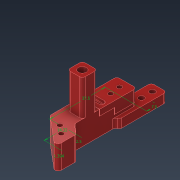
# Autodesk Inventor part: CH_01_0025_end_switch_mount
Saved by Autodesk Inventor 2022.3 (Build 263350030, 350C)
## iProperties
Created: 2022-03-07
Part Number: CH_01_0025_end_switch_mount
Material: Generic
Document SubType Name: Modeling
Designer: Tomasz Krakowski
Density: 1 g/cm^3
Appearance: Czerwona
Mass: 3.3096 g
Surface Area: 18.0709 cm^2
Volume: 3.3096 cm^3
Author: Tomasz Krakowski
Autodesk Inventor part; units mm, degrees
ref_plane "YZ Plane" through (0, 0, 0) normal (1, 0, 0) x (0, 1, 0)
ref_plane "XZ Plane" through (0, 0, 0) normal (0, 1, 0) x (-1, 0, 0)
ref_plane "XY Plane" through (0, 0, 0) normal (0, 0, 1) x (1, 0, 0)
sketch "Sketch2" plane through (0, 0, 0) normal (0, 1, 0) x (-1, 0, 0)
  line L0 (-10, 10) -> (-10, -10)
  line L1 (-10, -10) -> (10, -10)
  line L2 (10, -10) -> (10, -6.782)
  line L3 (10, -6.782) -> (-10, 10)
  line L4 (0, 0) -> (0, -10) construction
  line L5 (0, 0) -> (-10, 0) construction
  dimension "d7" = 20
  dimension "d8" = 20
  dimension "d15" = 50
  constraints: 12 end point, 4 perpendicular, 2 midpoint, 1 vertical
  measures "d7" distance of L0.end L1.end
  measures "d8" distance from line of L1 L0.start
  measures "d15" angle of L0 L3
extrude "Extrusion2" add sketch "Sketch2" along normal blind 16
sketch "Sketch4" plane through (0, 0, 0) normal (0, -1, 0) x (1, 0, 0)
  line L0 (6.2579, -0.3197) -> (-0.6365, -6.1048) construction
  line L1 (-10, -6.782) -> (10, 10) construction
  line L2 (6.2579, -0.3197) -> (2.7226, 3.8935) construction
  point P0 (0, 0)
  dimension "d29" = 9
  dimension "d30" = 5.5
  dimension "d43" = 9.5
  constraints: 4 end point, 2 coincident, 1 parallel, 1 perpendicular, 1 point on line
  measures "d29" distance of L0.start L0.end
  measures "d30" distance between parallel lines of L1 L0
  measures "d43" distance of L1.end L2.end
hole "Hole2" at (-0.6365, 0, -6.1048) at (6.2579, 0, -0.3197) direction (0, 1, 0) diameter 4.1 depth 7.5
sketch "Sketch5" plane through (0, 16, 0) normal (0, 1, 0) x (1, 0, 0)
  line L0 (10, -10) -> (10, 10) construction
  line L1 (10, 4.3595) -> (3.2779, 10)
  line L2 (10, 10) -> (-10, 10) construction
  line L3 (3.2779, 10) -> (10, 10)
  line L4 (10, 4.3595) -> (10, 10)
  line L5 (-10, 6.782) -> (10, -10) construction
  point P0 (0, 0)
  point P1 (10, -5.711)
  point P2 (-8, 10)
  point P3 (-9.2856, 6.1825)
  point P4 (6.7144, -7.2431)
  dimension "d39" = 11
  constraints: 6 end point, 2 point on line, 1 collinear, 1 parallel, 1 vertical
  measures "d39" distance between parallel lines of L1 L5
extrude "Extrusion3" cut sketch "Sketch5" against normal through all
sketch "Sketch3" plane through (0, 16, 0) normal (0, 1, 0) x (1, 0, 0)
  line L0 (-0.7246, -1.001) -> (1.8465, 2.0632) construction
  line L1 (4.5277, -0.1866) -> (-0.8346, 4.313) construction
  line L2 (-10, 6.782) -> (10, -10) construction
  point P0 (0, 0)
  dimension "d18" = 14
  dimension "d19" = 7
  dimension "d20" = 4
  constraints: 4 end point, 2 coincident, 2 perpendicular, 1 midpoint, 1 point on line
  measures "d18" distance from line of L2.end L0
  measures "d19" distance of L1.start L1.end
  measures "d20" distance between parallel lines of L2 L1
hole "Hole1" at (-0.8346, 16, -4.313) at (4.5277, 16, 0.1866) direction (0, -1, 0) diameter 3.1 depth 7.5
sketch "Sketch7" plane through (-10, 0, -10) normal (0, 0, -1) x (-1, 0, 0)
  line L0 (-13.2779, 16) -> (0, 16) projected
  line L1 (-13.2779, 16) -> (0, 16)
  line L2 (0, 16) -> (0, 0)
  line L3 (0, 0) -> (-13.2779, 0)
  line L4 (-13.2779, 0) -> (-13.2779, 16)
  point P0 (-10, 0)
  constraints: 8 end point, 2 parallel, 1 horizontal, 1 perpendicular
extrude "Extrusion4" add sketch "Sketch7" along normal blind 42
sketch "Sketch8" plane through (0, 16, 0) normal (0, 1, 0) x (1, 0, 0)
  line L0 (-3.1121, 47.03) -> (-2.2021, 40.0894) construction
  line L1 (3.2779, 10) -> (3.2779, 52) construction
  point P0 (0, 0)
  dimension "d50" = 5.48
  dimension "d51" = 6.39
  dimension "d52" = 7
  dimension "d53" = 4.97
  constraints: 2 end point
  measures "d50" distance from line of L1 L0.end
  measures "d51" distance from line of L1 L0.start
  measures "d52" distance of L0.start L0.end
  measures "d53" vertical distance of L0.start L1.end
sketch "Sketch9" plane through (0, 0, 0) normal (0, -1, 0) x (1, 0, 0)
  line L0 (3.2779, -10) -> (3.2779, -52) construction
  line L1 (3.2779, -38) -> (5.7779, -38)
  line L2 (5.7779, -38) -> (5.7779, -70)
  line L3 (5.7779, -70) -> (-4.7221, -70)
  line L4 (-4.7221, -70) -> (-4.7221, -52)
  line L5 (-10, -52) -> (3.2779, -52) construction
  line L6 (-4.7221, -52) -> (3.2779, -52)
  line L7 (3.2779, -52) -> (3.2779, -38)
  point P0 (0, 0)
  dimension "d61" = 14
  dimension "d62" = 2.5
  dimension "d63" = 8
  dimension "d64" = 18
  constraints: 12 end point, 4 perpendicular, 1 collinear, 1 horizontal, 1 point on line
  measures "d61" distance from line of L0.end L1
  measures "d62" distance between parallel lines of L2 L0
  measures "d63" distance from line of L0.end L4
  measures "d64" distance between parallel lines of L5 L3
extrude "Extrusion5" add sketch "Sketch9" against normal blind 6
sketch "Sketch10" plane through (0, 0, 0) normal (0, -1, 0) x (1, 0, 0)
  circle A0 centre (-0.6365, -6.1048) radius 2.05 construction
  line L0 (-0.6365, -6.1048) -> (0.7575, -6.1048) construction
  line L1 (0.7575, -6.1048) -> (0.7575, -65.4248) construction
  point P0 (0, 0)
  point P1 (-1.7425, -20.4248)
  point P2 (0.7575, -57.9248)
  dimension "d67" = 14.32
  dimension "d70" = 2.5
  dimension "d71" = 1.394
  dimension "d72" = 7.5
  dimension "d73" = 37.5
  constraints: 4 end point, 1 coincident, 1 horizontal, 1 point on line, 1 vertical
  measures "d67" distance from line of point (-1.742, -20.425) L0
  measures "d70" distance from line of L1 point (-1.742, -20.425)
  measures "d71" distance of L0.start L0.end
  measures "d72" distance of L1.end point (0.758, -57.925)
  measures "d73" vertical distance of point (0.758, -57.925) point (-1.742, -20.425)
hole "Hole4" at (0.7575, 0, -65.4248) at (0.7575, 0, -57.9248) direction (0, 1, 0) diameter 3.8 depth 8
hole "Hole5" at (-1.7425, 0, -20.4248) direction (0, 1, 0) diameter 5.5 depth 8
sketch "Sketch11" plane through (0, 16, 0) normal (0, 1, 0) x (1, 0, 0)
  line L0 (-6.7629, 15.4044) -> (3.2779, 15.4044)
  line L1 (3.2779, 15.4044) -> (3.2779, 25.4452)
  line L2 (3.2779, 25.4452) -> (-6.7629, 25.4452)
  line L3 (-6.7629, 25.4452) -> (-6.7629, 15.4044)
  line L4 (-6.7629, 15.4044) -> (3.2779, 25.4452) construction
  line L5 (3.2779, 15.4044) -> (-6.7629, 25.4452) construction
  line L6 (3.2779, 10) -> (3.2779, 52) construction
  circle A0 centre (-1.7425, 20.4248) radius 2.75 construction
  point P0 (0, 0)
  point P1 (-1.7425, 20.4248)
  constraints: 12 end point, 3 midpoint, 2 parallel, 2 perpendicular, 1 coincident, 1 collinear, 1 horizontal
extrude "Extrusion6" add sketch "Sketch11" along normal blind 24
sketch "Sketch12" plane through (3.2779, 0, -10) normal (1, 0, 0) x (0, 0, -1)
  line L0 (17, 16) -> (17, 12)
  line L1 (17, 12) -> (27, 12)
  line L2 (27, 12) -> (27, 8)
  line L3 (27, 8) -> (42, 8)
  line L4 (42, 16) -> (42, 6) construction
  line L5 (17, 16) -> (42, 16)
  line L6 (42, 16) -> (42, 8)
  point P0 (-10, 0)
  dimension "d90" = 4
  dimension "d91" = 15
  dimension "d92" = 10
  constraints: 12 end point, 4 perpendicular, 1 collinear, 1 parallel, 1 point on line, 1 vertical
  measures "d90" distance of L1.end L2.end
  measures "d91" distance between parallel lines of L4 L2
  measures "d92" distance from line of L1.end L0
extrude "Extrusion7" cut sketch "Sketch12" against normal through all
sketch "Sketch13" plane through (3.2779, 0, -10) normal (1, 0, 0) x (0, 0, -1)
  line L0 (17.2, 16) -> (42, 16)
  line L1 (42, 16) -> (42, 8)
  line L2 (42, 8) -> (27.2, 8)
  line L3 (27.2, 8) -> (27.2, 12)
  line L4 (27.2, 12) -> (17.2, 12)
  line L5 (17.2, 12) -> (17.2, 16)
  line L6 (27, 12) -> (17, 12) construction
  line L7 (27, 8) -> (27, 12) construction
  line L8 (42, 8) -> (42, 6) construction
  line L9 (15.4452, 16) -> (17, 16) construction
  point P0 (-10, 0)
  dimension "d95" = 0.2
  dimension "d96" = 0.2
  constraints: 12 end point, 4 perpendicular, 3 collinear
  measures "d95" distance from line of L6.end L5
  measures "d96" distance between parallel lines of L7 L3
extrude "Extrusion8" add sketch "Sketch13" against normal up to surface (13.2779 mm away) separate body
hole "Hole6" at (-2.2021, 16, -40.0894) at (-3.1121, 16, -47.03) direction (0, -1, 0) diameter 3.1 depth 8 bodies 2
sketch "Sketch14" plane through (3.2779, 16, -27.2) normal (0, 1, 0) x (1, 0, 0)
  line L0 (-3.6389, 4.646) -> (-9.6389, 4.646) construction
  line L1 (-3.6389, 6.546) -> (-9.6389, 6.546)
  line L2 (-9.6389, 2.746) -> (-3.6389, 2.746)
  arc A0 (-3.6389, 2.746) -> (-3.6389, 6.546) centre (-3.6389, 4.646) ccw
  arc A1 (-9.6389, 6.546) -> (-9.6389, 2.746) centre (-9.6389, 4.646) ccw
  line L3 (0, 0) -> (-13.2779, 0) construction
  line L4 (0, 9.8) -> (-13.2779, 9.8) construction
  line L5 (-6.6389, 9.8) -> (-6.6389, 4.646) construction
  line L6 (-6.6389, 4.646) -> (-6.6389, 0) construction
  point P0 (-3.2779, -27.2)
  dimension "d106" = 3.8
  dimension "d107" = 6
  constraints: 12 end point, 4 point on circle, 4 tangent, 3 midpoint, 2 centre point, 1 collinear, 1 parallel
  measures "d106" distance between parallel lines of L1 L2
  measures "d107" distance of L0.end L0.start
extrude "Extrusion9" cut sketch "Sketch14" against normal blind 2 bodies 2
sketch "Sketch15" plane through (3.2779, 14, -27.2) normal (0, 1, 0) x (1, 0, 0)
  arc A0 (-9.6389, 6.546) -> (-9.6389, 2.746) centre (-9.6389, 4.646) ccw construction
  line L0 (-3.6389, 2.746) -> (-9.6389, 2.746) construction
  arc A1 (-3.6389, 2.746) -> (-3.6389, 6.546) centre (-3.6389, 4.646) ccw construction
  line L1 (-9.6389, 6.546) -> (-3.6389, 6.546) construction
  line L2 (-3.6389, 4.646) -> (-9.6389, 4.646) construction
  line L3 (-3.6389, 5.746) -> (-9.6389, 5.746)
  line L4 (-9.6389, 3.546) -> (-3.6389, 3.546)
  arc A2 (-3.6389, 3.546) -> (-3.6389, 5.746) centre (-3.6389, 4.646) ccw
  arc A3 (-9.6389, 5.746) -> (-9.6389, 3.546) centre (-9.6389, 4.646) ccw
  point P0 (-3.2779, -27.2)
  point P1 (-6.6389, 4.646)
  dimension "d110" = 2.2
  constraints: 8 end point, 4 point on circle, 4 tangent, 2 centre point, 1 horizontal, 1 midpoint, 1 parallel
  measures "d110" distance between parallel lines of L3 L4
extrude "Extrusion10" cut sketch "Sketch15" against normal blind 2 bodies 2
sketch "Sketch16" plane through (3.2779, 12, -27) normal (0, 1, 0) x (1, 0, 0)
  line L0 (-9.6389, 5.946) -> (-3.6389, 5.946) construction
  line L1 (-6.6389, 5.946) -> (-6.6389, 3.746) construction
  line L2 (-9.6389, 3.746) -> (-3.6389, 3.746) construction
  point P0 (-3.2779, -27)
  point P1 (-6.6389, 4.846)
  point P2 (-6.6389, 4.846)
  constraints: 3 midpoint, 2 end point, 1 coincident
hole "Hole7" at (-3.3611, 12, -31.846) direction (0, -1, 0) diameter 3.1 depth 8 bodies 1
fillet "Fillet4" radius 2 17 edges at (-6.7629, 28, -15.4044) (3.2779, 28, -15.4044) (3.2779, 28, -25.4452) (-6.7629, 28, -25.4452) (10, 8, 10) (10, 8, -4.3595) (3.2779, 8, -10) (3.2779, 3, -38) (5.7779, 3, -38) (5.7779, 3, -70) (-4.7221, 3, -70) (-4.7221, 3, -52) (-10, 4, -52) (3.2779, 7, -52) (-10, 8, -6.782) (-10, 12, -52) (3.2779, 12, -52)
sketch "Sketch17" plane through (0, 40, 0) normal (0, 1, 0) x (1, 0, 0)
  point P0 (0, 0)
sketch "Sketch18" plane through (0, 40, 0) normal (0, 1, 0) x (1, 0, 0)
  line L0 (-6.7629, 23.4452) -> (-6.7629, 17.4044) construction
  line L1 (-6.7629, 20.4248) -> (-1.7425, 20.4248) construction
  line L2 (-1.7425, 20.4248) -> (-1.7425, 25.4452) construction
  line L3 (-4.7629, 25.4452) -> (1.2779, 25.4452) construction
  point P0 (0, 0)
  constraints: 4 end point, 2 midpoint, 2 perpendicular, 1 coincident
hole "Hole8" at (-1.7425, 40, -20.4248) direction (0, -1, 0) diameter 5.5 depth 12 bodies 1
equation "\"d96\" = d95"
body "Solid2"
body "Solid3"
